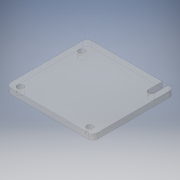
# Autodesk Inventor part: Halter_Tesla
Saved by Autodesk Inventor 2016 (Build 200138000, 138)
## iProperties
Created: 2018-06-04
Part Number: Halter_Tesla
Material: Polycarbonate, Clear
Document SubType Name: Modeling
Designer: Phil Erle
Density: 1.2 g/cm^3
Appearance: Polycarbonate - Clear
Author: Phil Erle
Autodesk Inventor part; units mm, degrees
ref_plane "YZ Plane" through (0, 0, 0) normal (1, 0, 0) x (0, 1, 0)
ref_plane "XZ Plane" through (0, 0, 0) normal (0, 1, 0) x (-1, 0, 0)
ref_plane "XY Plane" through (0, 0, 0) normal (0, 0, 1) x (1, 0, 0)
sketch "Sketch1" plane through (0, 0, 0) normal (0, 0, 1) x (1, 0, 0)
  line L0 (-37.5, -35) -> (37.5, -35)
  line L1 (37.5, -35) -> (37.5, 35)
  line L2 (37.5, 35) -> (-37.5, 35)
  line L3 (-37.5, 35) -> (-37.5, -35)
  line L4 (-37.5, -35) -> (37.5, 35) construction
  line L5 (37.5, -35) -> (-37.5, 35) construction
  point P0 (0, 0)
  dimension "d0" = 75
  dimension "d1" = 70
  constraints: 12 end point, 2 midpoint, 2 parallel, 1 horizontal, 1 perpendicular
  measures "d0" distance of L2.end L1.end
  measures "d1" distance of L1.end L0.end
extrude "Extrusion1" add sketch "Sketch1" along normal blind 5
sketch "Sketch2" plane through (0, 0, 5) normal (0, 0, 1) x (1, 0, 0)
  line L0 (-30, -30) -> (30, -30) construction
  line L1 (-37.5, -35) -> (37.5, -35) construction
  line L2 (-30, 23) -> (30, 23) construction
  point P0 (0, 0)
  point P1 (0, -30)
  dimension "d4" = 60
  dimension "d5" = 5
  dimension "d6" = 60
  dimension "d7" = 58
  dimension "d8" = 30
  constraints: 4 end point, 2 coincident, 2 horizontal, 1 midpoint, 1 vertical alignment
  measures "d4" distance of L0.start L0.end
  measures "d5" distance from line of L1 point (0, -30)
  measures "d6" distance of L2.start L2.end
  measures "d7" distance between parallel lines of L1 L2
  measures "d8" horizontal distance of point (0, 0) L2.end
hole "Hole1" at (-30, -30, 5) at (30, -30, 5) at (30, 23, 5) at (-30, 23, 5) direction (0, 0, -1) diameter 5.5 depth 8 tip angle 118 clearance for "Countersunk Flat Head Screw DIN EN ISO 2009" size "M5" standard "DIN"
fillet "Fillet1" radius 4 4 edges at (-37.5, 35, 2.5) (37.5, 35, 2.5) (-37.5, -35, 2.5) (37.5, -35, 2.5)
sketch "Sketch3" plane through (0, 0, 5) normal (0, 0, 1) x (1, 0, 0)
  circle A0 centre (30, 23) radius 2.75 projected
  line L0 (27.25, 23) -> (27.25, 35)
  line L1 (33.5, 35) -> (-33.5, 35) projected
  line L2 (32.75, 23) -> (32.75, 35)
  line L3 (32.75, 35) -> (27.25, 35)
  line L4 (32.75, 23) -> (27.25, 23)
  point P0 (0, 0)
  constraints: 8 end point, 2 point on circle, 2 vertical, 1 collinear, 1 parallel, 1 point on line
extrude "Extrusion2" cut sketch "Sketch3" against normal blind 5 contours A0 L0 L1 L2
body "Solid1"
